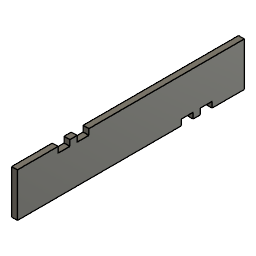
Laterales intermedio 1-2 piso (Autodesk Fusion 360 design; units mm, degrees)
Autodesk Fusion 360 part; units mm, degrees
sketch "Boceto1" plane through (0, 0, 0) normal (0, 1, 0) x (1, 0, 0)
  line L0 (-76.6693, 30.4647) -> (-76.6693, -124.8933)
  line L1 (-95, 0) -> (105, 0) construction
  line L2 (-76.6693, 30.4647) -> (-72.6693, 30.4647)
  line L3 (-72.6693, 30.4647) -> (-72.6693, -124.8933)
  line L4 (-76.6693, -124.8933) -> (-72.6693, -124.8933)
  dimension "d59" = 4
  constraint perpendicular L0 L2
  constraint perpendicular L2 L3
  constraint perpendicular L0 L4
  measures "d59" distance of L0 L3
extrude "Extruir1" add sketch "Boceto1" along normal blind 30
sketch "Boceto2" plane through (-72.6693, 0, 0) normal (1, 0, 0) x (0, 0, -1)
  line L0 (-124.8933, 0) -> (30.4647, 0)
  line L1 (30.4647, 0) -> (30.4647, 30)
  line L2 (30.4647, 30) -> (-124.8933, 30)
  line L3 (-124.8933, 30) -> (-124.8933, 0)
  line L4 (-76, 30) -> (-84, 30)
  line L5 (-84, 26) -> (-76, 26)
  line L6 (-76, 26) -> (-76, 30)
  line L7 (-89, 30) -> (-97, 30)
  line L8 (-97, 30) -> (-97, 28)
  line L9 (-89, 28) -> (-89, 30)
  line L10 (-97, 26) -> (-89, 26)
  line L11 (-89, 26) -> (-89, 30)
  line L12 (-76, 30) -> (-84, 30)
  line L13 (-97, 30) -> (-97, 26)
  line L14 (8.3256, 0) -> (0.3256, 0)
  line L15 (0.3256, 0) -> (0.3256, 4)
  line L16 (0.3256, 4) -> (8.3256, 4)
  line L17 (8.3256, 4) -> (8.3256, 0)
  line L18 (-4.6744, 0) -> (-12.6744, 0)
  line L19 (-12.6744, 0) -> (-12.6744, 4)
  line L20 (-12.6744, 4) -> (-4.6744, 4)
  line L21 (-4.6744, 4) -> (-4.6744, 0)
  line L22 (-84, 30) -> (-84, 26)
  dimension "d43" = 8
  dimension "d46" = 8
  dimension "d47" = 4
  dimension "d50" = 4
  dimension "d51" = 8
  dimension "d52" = 5
  dimension "d53" = 4
  dimension "d54" = 5
  dimension "d55" = 8
  dimension "d56" = 8
  dimension "d57" = 4
  constraint horizontal L4
  constraint horizontal L5
  constraint vertical L6
  constraint coincident L2 L4.start
  constraint horizontal L7
  constraint vertical L8
  constraint vertical L9
  constraint coincident L2 L7.start
  constraint horizontal L12
  constraint vertical L13
  constraint horizontal L10
  constraint vertical L11
  constraint horizontal L14
  constraint vertical L15
  constraint horizontal L16
  constraint vertical L17
  constraint coincident L0 L14.start
  constraint horizontal L18
  constraint vertical L19
  constraint horizontal L20
  constraint vertical L21
  constraint coincident L0 L18.start
  constraint perpendicular L5 L22
  measures "d43" distance of L8.end L9.start
  measures "d46" distance of L10.end L10.start
  measures "d47" distance of L4.start L5.end
  measures "d50" distance of L7 L10
  measures "d51" distance of L5.start L5.end
  measures "d52" distance of L11 L22
  measures "d53" distance of L14.start L16.end
  measures "d54" distance of L15 L21
  measures "d55" distance of L15.end L16.end
  measures "d56" distance of L19.end L20.end
  measures "d57" distance of L18.end L19.end
extrude "Extruir2" cut sketch "Boceto2" against normal through all contours L0 L18 L19 L20 L21 | L2 L7 L8 L9 L10 L11 L13 | L0 L14 L15 L16 L17 | L2 L4 L5 L6 L12 L22
sketch "Boceto3" plane through (-72.6693, 0, 0) normal (1, 0, 0) x (0, 0, -1)
  line L0 (-12.6744, 0) -> (-12.6744, 4)
  line L1 (-12.6744, 4) -> (-4.6744, 4)
  line L2 (-4.6744, 4) -> (-4.6744, 0)
  line L3 (-4.6744, 0) -> (0.3256, 0)
  line L4 (0.3256, 0) -> (0.3256, 4)
  line L5 (0.3256, 4) -> (8.3256, 4)
  line L6 (8.3256, 4) -> (8.3256, 0)
  line L7 (8.3256, 0) -> (30.4647, 0)
  line L8 (30.4647, 0) -> (30.4647, 30)
  line L9 (30.4647, 30) -> (-76, 30)
  line L10 (-76, 30) -> (-76, 26)
  line L11 (-76, 26) -> (-84, 26)
  line L12 (-84, 26) -> (-84, 30)
  line L13 (-84, 30) -> (-89, 30)
  line L14 (-89, 30) -> (-89, 26)
  line L15 (-89, 26) -> (-97, 26)
  line L16 (-97, 26) -> (-97, 30)
  line L17 (-97, 30) -> (-124.8933, 30)
  line L18 (-124.8933, 30) -> (-124.8933, 0)
  line L19 (-124.8933, 0) -> (-12.6744, 0)
  line L20 (-4.6744, 0) -> (-4.6744, 4)
  line L21 (-4.6744, 4) -> (-12.6744, 4)
  line L22 (-12.6744, 4) -> (-12.6744, 0)
  line L23 (-97, 30) -> (-97, 26)
  line L24 (-97, 26) -> (-89, 26)
  line L25 (-89, 26) -> (-89, 30)
  line L26 (8.3256, 0) -> (8.3256, 4)
  line L27 (8.3256, 4) -> (0.3256, 4)
  line L28 (0.3256, 4) -> (0.3256, 0)
  line L29 (-84, 30) -> (-84, 26)
  line L30 (-84, 26) -> (-76, 26)
  line L31 (-76, 26) -> (-76, 30)
  line L32 (30.4647, 0) -> (8.3256, 0)
  line L33 (0.3256, 0) -> (-4.6744, 0)
  line L34 (-97, 30) -> (-124.8933, 30)
  line L35 (30.4647, 30) -> (-76, 30)
  line L36 (30.4647, 0) -> (30.4647, 30)
  line L37 (-124.8933, 0) -> (-124.8933, 30)
  line L38 (-12.6744, 0) -> (-124.8933, 0)
  line L39 (-84, 30) -> (-89, 30)
